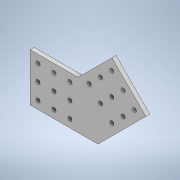
# Autodesk Inventor part: 3x3 V plate
Saved by Autodesk Inventor 2020 (Build 240168000, 168)
## iProperties
Created: 2020-01-28
Part Number: 3x3 V plate
Material: Generic
Document SubType Name: Modeling
Designer: 339294
Density: 1 g/cm^3
Appearance: Default
Author: 339294
Autodesk Inventor part; units mm, degrees
ref_plane "YZ Plane" through (0, 0, 0) normal (1, 0, 0) x (0, 1, 0)
ref_plane "XZ Plane" through (0, 0, 0) normal (0, 1, 0) x (-1, 0, 0)
ref_plane "XY Plane" through (0, 0, 0) normal (0, 0, 1) x (1, 0, 0)
sketch "Sketch1" plane through (0, 0, 0) normal (0, 0, 1) x (1, 0, 0)
  line L0 (76.2, 76.2) -> (0, 76.2)
  line L1 (0, 76.2) -> (0, 0)
  line L2 (76.2, 76.2) -> (130.0815, 130.0815)
  line L3 (130.0815, 130.0815) -> (183.9631, 76.2)
  line L4 (0, 0) -> (107.7631, 0)
  line L5 (183.9631, 76.2) -> (107.7631, 0)
  circle A0 centre (12.7, 12.7) radius 3.2512
  circle A1 centre (12.7, 38.1) radius 3.2512
  circle A2 centre (12.7, 63.5) radius 3.2512
  circle A3 centre (38.1, 12.7) radius 3.2512
  circle A4 centre (38.1, 38.1) radius 3.2512
  circle A5 centre (38.1, 63.5) radius 3.2512
  circle A6 centre (63.5, 12.7) radius 3.2512
  circle A7 centre (63.5, 38.1) radius 3.2512
  circle A8 centre (63.5, 63.5) radius 3.2512
  circle A9 centre (166.0026, 76.2) radius 3.2512
  circle A10 centre (148.042, 94.1605) radius 3.2512
  circle A11 centre (130.0815, 112.121) radius 3.2512
  circle A12 centre (148.042, 58.2395) radius 3.2512
  circle A13 centre (130.0815, 76.2) radius 3.2512
  circle A14 centre (112.121, 94.1605) radius 3.2512
  circle A15 centre (130.0815, 40.279) radius 3.2512
  circle A16 centre (112.121, 58.2395) radius 3.2512
  circle A17 centre (94.1605, 76.2) radius 3.2512
  dimension "d5" = 76.2
  dimension "d7" = 76.2
  dimension "d8" = 135
  dimension "d11" = 76.2
  dimension "d12" = 76.2
  dimension "d13" = 76.2
  dimension "d14" = 6.5024
  dimension "d15" = 12.7
  dimension "d16" = 12.7
  dimension "d19" = 25.4
  dimension "d22" = 25.4
  dimension "d25" = 6.5024
  dimension "d26" = 12.7
  dimension "d27" = 12.7
  dimension "d30" = 25.4
  dimension "d33" = 25.4
  constraints: 18 centre point, 12 end point, 3 perpendicular, 2 horizontal, 1 vertical, 34 other
  measures "d5" distance of L0.start L2.end
  measures "d7" distance of L2.end L3.end
  measures "d8" angle of L0 L2
  measures "d11" horizontal distance of L3.end L4.end
  measures "d12" distance of L0.start L0.end
  measures "d13" distance of L0.end L1.end
  measures "d14" diameter of A0
  measures "d15" distance from line of L4 A0.centre
  measures "d16" distance from line of L1 A0.centre
  measures "d19" distance of A0.centre A1.centre
  measures "d22" distance of A0.centre A3.centre
  measures "d25" diameter of A9
  measures "d26" distance from line of L5 A9.centre
  measures "d27" distance from line of L3 A9.centre
  measures "d30" distance of A9.centre A10.centre
  measures "d33" distance of A9.centre A12.centre
extrude "Extrusion1" add sketch "Sketch1" along normal blind 6.35
body "Solid1"
